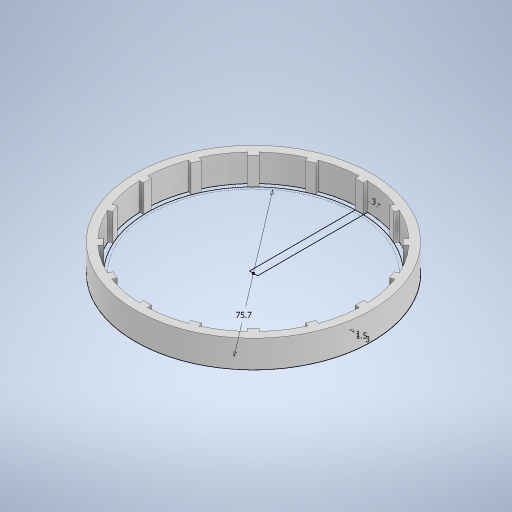
# Autodesk Inventor part: STI Hybrid 98 Cooling Shroud Lower Section Prototype
Saved by Autodesk Inventor 2023 (Build 270158000, 158)
## iProperties
Created: 2024-05-02
Part Number: STI Hybrid 98 Cooling Shroud Lower Section Prototype
Material: Generic
Document SubType Name: Modeling
Designer: incep
Density: 1 g/cm^3
Appearance: Default
Author: incep
## iProperties of the stored document STI Hybrid 98 Cooling Shroud Lower Section Prototype_3DPrint.ipt
Created: 2024-05-02
Part Number: STI Hybrid 98 Cooling Shroud Lower Section Prototype_3DPrint
Material: Generic
Document SubType Name: Modeling
Designer: incep
Density: 1 g/cm^3
Appearance: Default
Author: incep
Autodesk Inventor part; units mm, degrees
ref_plane "YZ Plane" through (0, 0, 0) normal (1, 0, 0) x (0, 1, 0)
ref_plane "XZ Plane" through (0, 0, 0) normal (0, 1, 0) x (-1, 0, 0)
ref_plane "XY Plane" through (0, 0, 0) normal (0, 0, 1) x (1, 0, 0)
sketch "Sketch1" plane through (0, 0, 0) normal (0, 1, 0) x (-1, 0, 0)
  circle A0 centre (0, 0) radius 37.85 construction
  circle A1 centre (0, 0) radius 38.85
  circle A2 centre (0, 0) radius 40.35
  circle A3 centre (0, 0) radius 43.35
  line L0 (1.5, -43.35) -> (-1.5, -43.35)
  line L1 (-1.5, -43.35) -> (-1.5, 0)
  line L2 (-1.5, 0) -> (1.5, 0)
  line L3 (1.5, 0) -> (1.5, -43.35)
  point P0 (0, -43.35)
  point P1 (1.5, -40.3221)
  point P2 (1.5, -38.821)
  point P3 (-1.5, -38.821)
  point P4 (-1.5, -40.3221)
  dimension "d0" = 75.7
  dimension "d1" = 1
  dimension "d2" = 1.5
  dimension "d3" = 3
  dimension "d4" = 3
  constraints: 8 end point, 3 centre point, 2 coincident, 2 midpoint, 2 parallel, 2 vertical alignment, 1 horizontal, 1 perpendicular, 2 other
  measures "d0" diameter of A0
  measures "d1" radial gap between concentric circles of A0 A1
  measures "d2" radial gap between concentric circles of A1 A2
  measures "d4" distance of L0.start L0.end
extrude "Extrusion1" add sketch "Sketch1" along normal blind 10 contours L1 A3 L3 A2 | A2 L3 A3 L1
extrude "Extrusion2" add sketch "Sketch1" along normal blind 10 contours A1 L3 A2 L1 picked at (1.1667, -39.33)
pattern_circular "Circular Pattern1" count 16 over 360 about axis through (0, -10, 0) along (0, 1, 0) of "Extrusion2"
body "Solid1"
